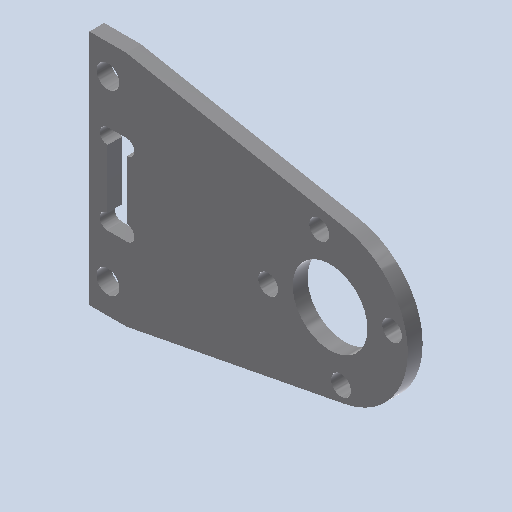
# Autodesk Inventor part: Shoulder_side_frame
Saved by Autodesk Inventor 2022.4 (Build 264492000, 492)
## iProperties
Created: 2016-05-05
Part Number: Shoulder_side_frame
Material: アルミニウム 2014-T4
Document SubType Name: Modeling
Designer: hiroaki
Density: 2.8 g/cm^3
Appearance: 滑らか - 淡い灰色
Mass: 5.10167 g
Surface Area: 23.2279 cm^2
Volume: 1.82202 cm^3
Description: A2017 T2
Author: hiroaki
Autodesk Inventor part; units mm, degrees
ref_plane "YZ Plane" through (0, 0, 0) normal (1, 0, 0) x (0, 1, 0)
ref_plane "XZ Plane" through (0, 0, 0) normal (0, 1, 0) x (-1, 0, 0)
ref_plane "XY Plane" through (0, 0, 0) normal (0, 0, 1) x (1, 0, 0)
sketch "スケッチ1" plane through (0, 0, 0) normal (0, 0, 1) x (1, 0, 0)
  circle A0 centre (-1.476, 8.3709) radius 1.35
  circle A1 centre (0, 0) radius 5.05
  line L0 (-30, 6) -> (-27.5, 6) construction
  line L1 (-27.5, 6) -> (-27.5, -6) construction
  line L2 (-27.5, -6) -> (-30, -6) construction
  line L3 (-30, -6) -> (-30, 6) construction
  line L4 (-27.45, 6.05) -> (-30.05, 6.05) construction
  line L5 (-30.05, 6.05) -> (-30.05, -6.05) construction
  line L6 (-30.05, -6.05) -> (-27.45, -6.05) construction
  line L7 (-27.45, -6.05) -> (-27.45, 6.05) construction
  circle A2 centre (-30.05, 5) radius 1.05 construction
  line L8 (-27.45, 6.05) -> (-30.05, 6.05)
  arc A3 (-30.05, 6.05) -> (-30.05, 3.95) centre (-30.05, 5) ccw
  line L9 (-30.05, 3.95) -> (-30.05, -3.95)
  line L10 (-28.75, 6.05) -> (-28.75, -6.05) construction
  line L11 (-30.05, 0) -> (-27.5, 0) construction
  arc A4 (-30.05, -3.95) -> (-30.05, -6.05) centre (-30.05, -5) ccw
  line L12 (-30.05, -6.05) -> (-27.45, -6.05)
  line L13 (-27.45, 3.95) -> (-27.45, -3.95)
  arc A5 (-27.45, 3.95) -> (-27.45, 6.05) centre (-27.45, 5) ccw
  arc A6 (-27.45, -6.05) -> (-27.45, -3.95) centre (-27.45, -5) ccw
  circle A7 centre (-30, 12) radius 1.55
  circle A8 centre (-30, -12) radius 1.55
  line L14 (-32.5, 16) -> (-27.5, 16)
  line L15 (-32.5, -16) -> (-27.5, -16)
  arc A9 (1.9894, -10.3098) -> (1.9894, 10.3098) centre (0, 0) ccw
  line L16 (-32.5, 16) -> (-32.5, -16)
  line L17 (-27.5, 16) -> (1.9894, 10.3098)
  line L18 (1.9894, -10.3098) -> (-27.5, -16)
  line L19 (-1.476, 8.3709) -> (0, 0) construction
  line L20 (0, 10.6937) -> (0, -10.6937) construction
  circle A10 centre (-8.3709, -1.476) radius 1.35
  circle A11 centre (1.476, -8.3709) radius 1.35
  circle A12 centre (8.3709, 1.476) radius 1.35
  point P0 (-28.775, 0)
  dimension "d29" = 2.1
  dimension "d4" = 2.7
  dimension "d9" = 10.1
  dimension "d10" = 2.5
  dimension "d30" = 0.05
  dimension "d31" = 6
  dimension "d33" = 3.1
  dimension "d57" = 32
  dimension "d61" = 32.5
  dimension "d62" = 5
  dimension "d63" = 2.5
  dimension "d65" = 10
  dimension "d66" = 10.5
  dimension "d67" = 8.5
  dimension "d69" = 10
  dimension "d72" = 360
  constraints: 42 end point, 12 centre point, 10 point on circle, 6 midpoint, 5 parallel, 5 symmetric about line, 5 tangent, 4 coincident, 4 perpendicular, 3 horizontal, 3 point on line, 3 vertical, 3 vertical alignment, 2 collinear, 2 equal radius, 1 horizontal alignment, 16 other
  measures "d4" diameter of A0
  measures "d9" diameter of A1
  measures "d10" distance of L0.start L0.end
  measures "d30" distance between parallel lines of L4 L0
  measures "d31" distance from line of L0 A7.centre
  measures "d33" diameter of A7
  measures "d57" distance of L15.start L14.start
  measures "d61" distance from line of point (0, 0) L16
  measures "d62" distance of L14.start L14.end
  measures "d63" horizontal distance of L14.start A7.centre
  measures "d65" distance between parallel lines of L14 L0
  measures "d66" radius of A9
  measures "d67" distance of L19.start L19.end
  measures "d69" angle of L20 L19
extrude "押し出し1" add sketch "スケッチ1" along normal blind 2
equation "\"d23\" = 7"
